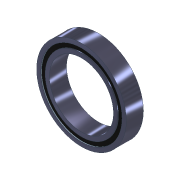
# Autodesk Inventor part: 6702ZZ-bearing-15x21x4
Saved by Autodesk Inventor 2020 (Build 240168000, 168)
## iProperties
Created: 2016-09-14
Part Number: 6702ZZ-bearing-15x21x4
Material: Generic
Document SubType Name: Modeling
Designer: Kostic
Density: 1 g/cm^3
Appearance: Steel Blue
Author: Kostic
Autodesk Inventor part; units mm, degrees
ref_plane "YZ Plane" through (0, 0, 0) normal (1, 0, 0) x (0, 1, 0)
ref_plane "XZ Plane" through (0, 0, 0) normal (0, 1, 0) x (-1, 0, 0)
ref_plane "XY Plane" through (0, 0, 0) normal (0, 0, 1) x (1, 0, 0)
sketch "Sketch1" plane through (0, 0, 0) normal (0, 0, 1) x (1, 0, 0)
  line L0 (0, 0) -> (0, 10) construction
  line L1 (0, 0) -> (10, 0) construction
  line L2 (7.5, 2) -> (8.5, 2)
  line L3 (8.5, 2) -> (8.5, -2)
  line L4 (8.5, -2) -> (7.5, -2)
  line L5 (7.5, -2) -> (7.5, 2)
  line L6 (8.5, 1.8) -> (9.5, 1.8)
  line L7 (9.5, 1.8) -> (9.5, -1.8)
  line L8 (9.5, -1.8) -> (8.5, -1.8)
  line L9 (8.5, -1.8) -> (8.5, 1.8)
  line L10 (9.5, 2) -> (10.5, 2)
  line L11 (10.5, 2) -> (10.5, -2)
  line L12 (10.5, -2) -> (9.5, -2)
  line L13 (9.5, -2) -> (9.5, 2)
  line L14 (8.5, 1.3) -> (9.5, 1.3)
  line L15 (8.5, -1.3) -> (9.5, -1.3)
  line L16 (8.52, 4.2678) -> (8.52, -4.334) construction
  line L17 (9.48, 3.8746) -> (9.48, -4.06) construction
  circle A0 centre (9, 0) radius 0.48
  point P0 (8.5, 1.3)
  dimension "d0" = 10
  dimension "d1" = 90
  dimension "d2" = 1
  dimension "d3" = 4
  dimension "d5" = 3.6
  dimension "d6" = 0.2
  dimension "d7" = 2
  dimension "d8" = 1
  dimension "d9" = 4
  dimension "d10" = 7.5
  dimension "d11" = 2
  dimension "d13" = 10.5
  dimension "d14" = 0.5
  dimension "d15" = 0.5
  dimension "d16" = 0.02
  dimension "d17" = 0.02
  constraints: 36 end point, 6 parallel, 6 perpendicular, 6 point on line, 4 horizontal, 3 vertical, 2 tangent, 1 centre point, 1 collinear
  measures "d0" distance of L0.start L0.end
  measures "d1" angle of L1 L0
  measures "d2" distance of L3.end L4.end
  measures "d3" distance of L2.end L3.end
  measures "d5" distance of L6.end L7.end
  measures "d6" distance between parallel lines of L2 L6
  measures "d7" distance from line of L0.start L2
  measures "d8" distance of L11.end L12.end
  measures "d9" distance of L10.end L11.end
  measures "d10" distance from line of L0.start L5
  measures "d11" distance from line of L0.start L10
  measures "d13" distance from line of L0.start L11
  measures "d14" distance between parallel lines of L8 L15
  measures "d15" distance between parallel lines of L14 L6
  measures "d16" distance between parallel lines of L9 L16
  measures "d17" distance between parallel lines of L7 L17
revolve "Revolution1" add sketch "Sketch1" angle 360 about axis through (0, 0, 0) along (0, 1, 0) contours L2 L3 L4 L5 | L6 L7 L14 L3 | L13 L10 L11 L12 L7 | L3 L15 L7 L8 | A0
equation "\"d5\" = d9 - 2 * d6"
equation "\"d7\" = 0.5 * d3"
equation "\"d8\" = d2"
equation "\"d9\" = d3"
equation "\"d11\" = d7"
equation "\"d17\" = d16"
body "Solid1"
